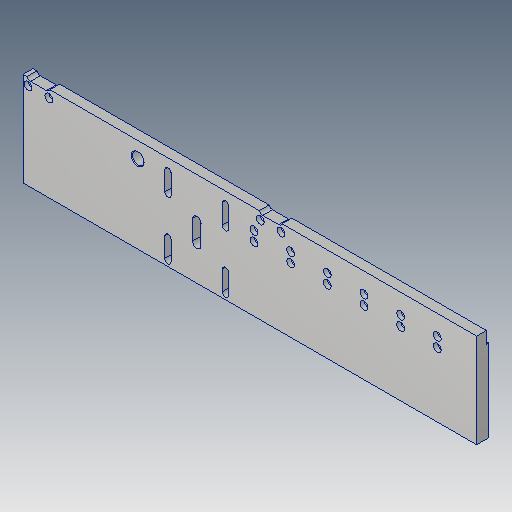
# Autodesk Inventor part: Frame Back
Saved by Autodesk Inventor 2019 (Build 230136000, 136)
## iProperties
Created: 2019-01-21
Part Number: Frame Back
Material: Aluminum 6061
Document SubType Name: Modeling
Designer: LillaHunden
Density: 2.7 g/cm^3
Appearance: Aluminum - Flat
Author: LillaHunden
Autodesk Inventor part; units mm, degrees
ref_plane "YZ Plane" through (0, 0, 0) normal (1, 0, 0) x (0, 1, 0)
ref_plane "XZ Plane" through (0, 0, 0) normal (0, 1, 0) x (-1, 0, 0)
ref_plane "XY Plane" through (0, 0, 0) normal (0, 0, 1) x (1, 0, 0)
sketch "Sketch1" plane through (0, 0, 0) normal (0, 0, 1) x (1, 0, 0)
  line L0 (-165.2266, -26.9823) -> (205.7734, -26.9823)
  line L1 (205.7734, -26.9823) -> (205.7734, -103.9647)
  line L2 (205.7734, -103.9647) -> (-165.2266, -103.9647)
  line L3 (-165.2266, -103.9647) -> (-165.2266, -26.9823)
  line L4 (15.7734, -103.9647) -> (41.2734, -103.9647) construction
  point P0 (0, 0)
  point P1 (20.2734, -103.9647)
  constraints: 8 end point, 2 parallel, 1 horizontal, 1 horizontal alignment, 1 midpoint, 1 perpendicular
extrude "Extrusion1" add sketch "Sketch1" along normal blind 10
sketch "Sketch2" plane through (-165.2266, -103.9647, 0) normal (-1, 0, 0) x (0, 0, 1)
  line L0 (0, 0) -> (0, 76.9823) construction
  line L1 (0, 0) -> (10, 0) projected
  line L2 (10, 76.9823) -> (10, 0) construction
  line L3 (0, 76.9823) -> (10, 76.9823) construction
  line L4 (2, 67) -> (-282, 67) construction
  line L5 (2, 67) -> (2, 76.9823) construction
  line L6 (-282, 76.9823) -> (2, 76.9823) construction
  line L7 (0, 103.9647) -> (2, 103.9647)
  line L8 (2, 103.9647) -> (2, 67)
  line L9 (2, 67) -> (0, 67)
  line L10 (0, 67) -> (0, 103.9647)
  line L11 (-282, 76.9823) -> (-282, 67) projected
  constraints: 8 end point, 2 parallel, 1 horizontal, 1 perpendicular, 1 other
extrude "Extrusion2" cut sketch "Sketch2" against normal through all
sketch "Sketch3" plane through (0, 0, 0) normal (0, 0, -1) x (-1, 0, 0)
  circle A0 centre (71.5266, -39.9823) radius 2.5 construction
  arc A1 (66.419, -43.1308) -> (56.0091, -36.9647) centre (56.0091, -48.8349) ccw
  line L0 (165.2266, -36.9647) -> (-205.7734, -36.9647) construction
  line L1 (71.5266, -34.9823) -> (71.5266, -45.9823) construction
  arc A2 (87.044, -36.9647) -> (76.6341, -43.1308) centre (87.044, -48.8349) ccw
  line L2 (56.0091, -36.9647) -> (87.044, -36.9647)
  arc A3 (66.419, -43.1308) -> (76.6341, -43.1308) centre (71.5266, -39.9823) ccw
  arc A4 (75.5133, -36.9647) -> (67.5399, -36.9647) centre (71.5266, -39.9823) ccw construction
  point P0 (0, 0)
  dimension "d9" = 6
  constraints: 10 point on circle, 5 centre point, 4 end point, 3 point on line, 3 symmetric about line, 2 tangent, 1 coincident, 1 collinear, 1 other
  measures "d9" radius of A3
extrude "Extrusion3" cut sketch "Sketch3" against normal up to surface (2 mm away)
sketch "Sketch4" plane through (0, 0, 0) normal (0, 0, -1) x (-1, 0, 0)
  circle A0 centre (23.2266, -67.9647) radius 18.9 projected
  circle A1 centre (23.2266, -67.9647) radius 19.5 projected
  point P0 (0, 0)
extrude "Extrusion4" cut sketch "Sketch4" against normal blind 3 contours A0 | A1
sketch "Sketch5" plane through (-23.2266, -67.9647, 3) normal (0, 0, -1) x (-1, 0, 0)
  circle A0 centre (0, 0) radius 2.5 projected
  circle A1 centre (0, 0) radius 3.5
  point P0 (-23.2266, 67.9647)
  dimension "d15" = 1
  constraints: 1 centre point
  measures "d15" radial gap between concentric circles of A0 A1
extrude "Extrusion5" cut sketch "Sketch5" against normal through all contours A0 | A1
sketch "Sketch6" plane through (0, 0, 0) normal (0, 0, -1) x (-1, 0, 0)
  circle A0 centre (-0.3434, -44.3947) radius 2.6 projected
  circle A1 centre (46.7966, -44.3947) radius 2.6 projected
  circle A2 centre (46.7966, -91.5347) radius 2.6 projected
  circle A3 centre (-0.3434, -91.5347) radius 2.6 projected
  point P0 (0, 0)
hole "Hole1" at (0.3434, -91.5347, 0) at (-46.7966, -91.5347, 0) at (0.3434, -44.3947, 0) at (-46.7966, -44.3947, 0) direction (0, 0, 1) diameter 4.134 depth 14.2 thread size "M5x0.8" class "6H" standard "ISO Metric profile"
chamfer "Chamfer3" distance 0.2 angle 45 8 edges at (0.3434, -46.4617, 10) (-46.7966, -46.4617, 10) (-46.7966, -93.6017, 10) (0.3434, -93.6017, 10) (0.3434, -93.6017, 0) (-46.7966, -93.6017, 0) (-46.7966, -46.4617, 0) (0.3434, -46.4617, 0)
sketch "Sketch7" plane through (-165.2266, -36.9647, 2) normal (0, 0, -1) x (-1, 0, 0)
  circle A0 centre (-93.7, -3.0177) radius 4.7625 projected
  circle A1 centre (-93.7, -3.0177) radius 4.7125
  point P0 (-165.2266, 36.9647)
  dimension "d31" = 0.05
  constraints: 1 centre point
  measures "d31" radial gap between concentric circles of A0 A1
extrude "Extrusion6" cut sketch "Sketch7" against normal through all contours A0 | A1
chamfer "Chamfer4" distance 0.5 angle 45 2 edges at (-66.7641, -39.9823, 2) (-66.7641, -39.9823, 10)
sketch "Sketch8" plane through (-165.2266, -36.9647, 2) normal (0, 0, -1) x (-1, 0, 0)
  line L0 (-18, 8.4823) -> (-7, 8.4823) construction
  line L1 (-7, 8.4823) -> (-7, 12.6239) construction
  line L2 (-18, 12.6239) -> (-18, 8.4823) construction
  line L3 (-19, 7.9823) -> (-6, 7.9823) projected
  line L4 (-19, 9.9823) -> (-19, 7.9823) projected
  line L5 (-6, 7.9823) -> (-6, 9.9823) projected
  arc A0 (-21.8284, 9.9823) -> (-19, 7.9823) centre (-19, 10.9823) ccw
  line L6 (-371, 9.9823) -> (0, 9.9823) projected
  line L7 (-21.8284, 9.9823) -> (-6, 9.9823)
  line L8 (-12.5, 7.9823) -> (-12.5, 13.9823)
  arc A1 (-6, 7.9823) -> (-3.1716, 9.9823) centre (-6, 10.9823) ccw
  line L9 (-3.1716, 9.9823) -> (-6, 9.9823)
  point P0 (-165.2266, 36.9647)
  dimension "d37" = 6
  constraints: 6 end point, 5 point on circle, 4 point on line, 2 centre point, 1 collinear, 1 midpoint, 1 perpendicular, 1 symmetric about line, 1 tangent, 1 vertical, 1 other
  measures "d37" diameter of A0
extrude "Extrusion7" cut sketch "Sketch8" against normal through all
sketch "Sketch9" plane through (-165.2266, -36.9647, 2) normal (0, 0, -1) x (-1, 0, 0)
  line L0 (-209, 9.9823) -> (-209, 7.9823) projected
  line L1 (-209, 7.9823) -> (-196, 7.9823) projected
  line L2 (-196, 7.9823) -> (-196, 9.9823) projected
  line L3 (-190, 9.9823) -> (-196, 9.9823) projected
  line L4 (-190, 0) -> (-190, 9.9823) projected
  line L5 (-215, 0) -> (-190, 0) projected
  line L6 (-215, 0) -> (-215, 9.9823) projected
  line L7 (-209, 9.9823) -> (-215, 9.9823) projected
  arc A0 (-211.8284, 9.9823) -> (-209, 7.9823) centre (-209, 10.9823) ccw
  line L8 (-202.5, 7.9823) -> (-202.5, 9.9823) construction
  arc A1 (-196, 7.9823) -> (-193.1716, 9.9823) centre (-196, 10.9823) ccw
  line L9 (-371, 9.9823) -> (-21.8284, 9.9823) projected
  line L10 (-211.8284, 9.9823) -> (-193.1716, 9.9823)
  point P0 (-165.2266, 36.9647)
  dimension "d40" = 6
  constraints: 5 end point, 5 point on circle, 3 point on line, 2 centre point, 2 midpoint, 1 symmetric about line, 1 tangent, 1 vertical, 1 other
  measures "d40" diameter of A0
extrude "Extrusion8" cut sketch "Sketch9" against normal through all contours L9 L2 L1 L0 | L0 A0 L7 | L3 A1 L2
sketch "Sketch10" plane through (0, 0, 0) normal (0, 0, -1) x (-1, 0, 0)
  circle A0 centre (23.2266, -67.9647) radius 3.5 construction
  line L0 (23.2266, -75.9647) -> (23.2266, -59.9647) construction
  line L1 (3.7266, -75.9647) -> (3.7266, -59.9647)
  line L2 (42.7266, -59.9647) -> (42.7266, -75.9647)
  arc A1 (3.7266, -75.9647) -> (42.7266, -75.9647) centre (23.2266, -75.9647) ccw
  arc A2 (42.7266, -59.9647) -> (3.7266, -59.9647) centre (23.2266, -59.9647) ccw
  circle A3 centre (23.2266, -67.9647) radius 3.5 construction
  circle A4 centre (23.2266, -67.9647) radius 19.5 construction
  line L3 (56.0091, -36.9647) -> (-205.7734, -36.9647) construction
  point P0 (0, 0)
  dimension "d43" = 8
  constraints: 8 end point, 5 tangent, 4 point on circle, 2 centre point, 1 midpoint, 1 parallel, 1 vertical
  measures "d43" distance of L0.end A0.centre
extrude "Extrusion9" cut sketch "Sketch10" against normal up to surface (3 mm away)
sketch "Sketch11" plane through (0, 0, 0) normal (0, 0, -1) x (-1, 0, 0)
  line L0 (-0.3434, -36.3947) -> (-0.3434, -52.3947) construction
  line L1 (-2.9434, -36.3947) -> (-2.9434, -52.3947)
  line L2 (2.2566, -52.3947) -> (2.2566, -36.3947)
  arc A0 (2.2566, -36.3947) -> (-2.9434, -36.3947) centre (-0.3434, -36.3947) ccw
  arc A1 (-2.9434, -52.3947) -> (2.2566, -52.3947) centre (-0.3434, -52.3947) ccw
  circle A2 centre (-0.3434, -44.3947) radius 2.067 construction
  circle A3 centre (46.7966, -44.3947) radius 2.267 construction
  line L3 (56.0091, -36.9647) -> (-205.7734, -36.9647) construction
  line L4 (46.7966, -36.3947) -> (46.7966, -52.3947) construction
  line L5 (44.1966, -36.3947) -> (44.1966, -52.3947)
  line L6 (49.3966, -52.3947) -> (49.3966, -36.3947)
  arc A4 (49.3966, -36.3947) -> (44.1966, -36.3947) centre (46.7966, -36.3947) ccw
  arc A5 (44.1966, -52.3947) -> (49.3966, -52.3947) centre (46.7966, -52.3947) ccw
  line L7 (-0.3434, -83.5347) -> (-0.3434, -99.5347) construction
  line L8 (-2.9434, -83.5347) -> (-2.9434, -99.5347)
  line L9 (2.2566, -99.5347) -> (2.2566, -83.5347)
  arc A6 (2.2566, -83.5347) -> (-2.9434, -83.5347) centre (-0.3434, -83.5347) ccw
  arc A7 (-2.9434, -99.5347) -> (2.2566, -99.5347) centre (-0.3434, -99.5347) ccw
  line L10 (46.7966, -83.5347) -> (46.7966, -99.5347) construction
  line L11 (44.1966, -83.5347) -> (44.1966, -99.5347)
  line L12 (49.3966, -99.5347) -> (49.3966, -83.5347)
  arc A8 (49.3966, -83.5347) -> (44.1966, -83.5347) centre (46.7966, -83.5347) ccw
  arc A9 (44.1966, -99.5347) -> (49.3966, -99.5347) centre (46.7966, -99.5347) ccw
  point P0 (0, 0)
  point P1 (46.7966, -44.3947)
  point P2 (46.7966, -44.3947)
  point P3 (-0.3434, -91.5347)
  point P4 (-0.3434, -91.5347)
  point P5 (46.7966, -91.5347)
  point P6 (46.7966, -91.5347)
  dimension "d46" = 8
  dimension "d47" = 5.2
  dimension "d50" = 47.14
  dimension "d53" = 47.14
  constraints: 32 end point, 16 point on circle, 8 centre point, 4 coincident, 4 tangent, 2 vertical, 1 collinear, 1 horizontal, 1 midpoint, 1 parallel, 38 other
  measures "d46" distance of point (-0.343, -44.395) L0.end
  measures "d47" diameter of A1
  measures "d50" distance of L1.start L5.start
  measures "d53" distance of L1.start L8.start
extrude "Extrusion10" cut sketch "Sketch11" against normal through all
sketch "Sketch12" plane through (0, 0, 3) normal (0, 0, -1) x (-1, 0, 0)
  circle A0 centre (23.2266, -67.9647) radius 3.5 construction
  line L0 (23.2266, -75.9647) -> (23.2266, -59.9647) construction
  circle A1 centre (23.2266, -67.9647) radius 3.5 construction
  line L1 (19.7266, -75.9647) -> (19.7266, -59.9647)
  line L2 (26.7266, -59.9647) -> (26.7266, -75.9647)
  arc A2 (19.7266, -75.9647) -> (26.7266, -75.9647) centre (23.2266, -75.9647) ccw
  arc A3 (26.7266, -59.9647) -> (19.7266, -59.9647) centre (23.2266, -59.9647) ccw
  point P0 (0, 0)
  dimension "d58" = 8
  constraints: 8 end point, 4 point on circle, 4 tangent, 2 centre point, 1 midpoint, 1 parallel, 1 vertical
  measures "d58" distance of A1.centre L0.end
extrude "Extrusion11" cut sketch "Sketch12" against normal through all
sketch "Sketch13" plane through (0, 0, 10) normal (0, 0, 1) x (1, 0, 0)
  line L0 (-146.2266, -26.9823) -> (-146.2266, -28.9823) construction
  line L1 (-146.2266, -28.9823) -> (-159.2266, -28.9823) construction
  line L2 (-159.2266, -28.9823) -> (-159.2266, -26.9823) construction
  line L3 (-165.2266, -26.9823) -> (-159.2266, -26.9823) construction
  line L4 (-165.2266, -36.9647) -> (-165.2266, -26.9823) construction
  line L5 (-140.2266, -36.9647) -> (-165.2266, -36.9647) construction
  line L6 (-140.2266, -36.9647) -> (-140.2266, -26.9823) construction
  line L7 (-146.2266, -26.9823) -> (-140.2266, -26.9823) construction
  line L8 (43.7734, -26.9823) -> (43.7734, -28.9823) construction
  line L9 (43.7734, -28.9823) -> (30.7734, -28.9823) construction
  line L10 (30.7734, -28.9823) -> (30.7734, -26.9823) construction
  line L11 (24.7734, -26.9823) -> (30.7734, -26.9823) construction
  line L12 (24.7734, -36.9647) -> (24.7734, -26.9823) construction
  line L13 (49.7734, -36.9647) -> (24.7734, -36.9647) construction
  line L14 (49.7734, -36.9647) -> (49.7734, -26.9823) construction
  line L15 (43.7734, -26.9823) -> (49.7734, -26.9823) construction
  circle A0 centre (-161.2266, -33.2125) radius 1.621 projected
  circle A1 centre (-144.2266, -33.2125) radius 1.621 projected
  point P0 (0, 0)
  point P1 (-161.2266, -33.2125)
  point P2 (-144.2266, -33.2125)
  point P3 (28.7734, -33.2125)
  point P4 (45.7734, -33.2125)
  dimension "d61" = 4
  dimension "d62" = 4
  dimension "d63" = 4
  dimension "d64" = 4
  constraints: 3 horizontal alignment
  measures "d61" distance from line of L4 point (-161.227, -33.213)
  measures "d62" distance from line of L6 point (-144.227, -33.213)
  measures "d63" distance from line of L12 point (28.773, -33.213)
  measures "d64" distance from line of L14 point (45.773, -33.213)
hole "Hole2" at (-161.2266, -33.2125, 10) at (-144.2266, -33.2125, 10) at (28.7734, -33.2125, 10) at (45.7734, -33.2125, 10) direction (0, 0, -1) diameter 3.4 depth 14.2 counterbore diameter 6.5 counterbore depth 3.4 clearance for "Socket Head Cap Screw ISO 4762" size "M3" standard "ISO"
sketch "Sketch14" plane through (0, 0, 10) normal (0, 0, 1) x (1, 0, 0)
  circle A0 centre (77.1068, -51.298) radius 1.621 construction
  circle A1 centre (173.6068, -51.298) radius 1.621 construction
  line L0 (108.2734, -36.9647) -> (108.2734, -41.9647) construction
  line L1 (108.2734, -41.9647) -> (93.2734, -41.9647) construction
  line L2 (93.2734, -41.9647) -> (93.2734, -36.9647) construction
  line L3 (12.7734, -36.9647) -> (93.2734, -36.9647) construction
  line L4 (12.7734, -55.9647) -> (12.7734, -36.9647) construction
  line L5 (205.7734, -55.9647) -> (12.7734, -55.9647) construction
  line L6 (205.7734, -55.9647) -> (205.7734, -36.9647) construction
  line L7 (108.2734, -36.9647) -> (205.7734, -36.9647) construction
  circle A2 centre (23.6068, -43.298) radius 1.621 projected
  circle A3 centre (53.6068, -51.298) radius 1.621 projected
  circle A4 centre (83.6068, -51.298) radius 1.621 projected
  circle A5 centre (113.6068, -43.298) radius 1.621 projected
  circle A6 centre (143.6068, -51.298) radius 1.621 projected
  circle A7 centre (173.6068, -43.298) radius 1.621 projected
  circle A8 centre (143.6068, -43.298) radius 1.621 projected
  circle A9 centre (113.6068, -51.298) radius 1.621 projected
  circle A10 centre (83.6068, -43.298) radius 1.621 projected
  circle A11 centre (53.6068, -43.298) radius 1.621 projected
  circle A12 centre (23.6068, -51.298) radius 1.621 projected
  point P0 (0, 0)
  point P1 (173.6068, -43.298)
  point P2 (143.6068, -51.298)
  point P3 (113.6068, -51.298)
  point P4 (83.6068, -51.298)
  point P5 (53.6068, -51.298)
  point P6 (23.6068, -51.298)
  point P7 (173.6068, -43.298)
  point P8 (143.6068, -43.298)
  point P9 (113.6068, -43.298)
  point P10 (83.6068, -43.298)
  point P11 (53.6068, -43.298)
  point P12 (23.6068, -43.298)
  dimension "d81" = 30
  dimension "d84" = 8
  constraints: 1 horizontal, 1 vertical, 11 other
  measures "d81" distance of A1.centre point (143.607, -51.298)
  measures "d84" distance of A1.centre point (173.607, -43.298)
hole "Hole3" at (173.6068, -43.298, 10) at (173.6068, -51.298, 10) at (143.6068, -51.298, 10) at (143.6068, -43.298, 10) at (113.6068, -51.298, 10) at (113.6068, -43.298, 10) at (83.6068, -43.298, 10) at (83.6068, -51.298, 10) at (53.6068, -51.298, 10) at (53.6068, -43.298, 10) at (23.6068, -51.298, 10) at (23.6068, -43.298, 10) direction (0, 0, -1) diameter 3.242 depth 11.8 counterbore diameter 6.5 counterbore depth 3.4 thread size "M4x0.7" class "6H" standard "ISO Metric profile"
body "Solid1"
